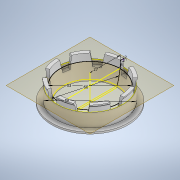
# Autodesk Inventor part: motor_frontalholder
Saved by Autodesk Inventor 2020 (Build 240168000, 168)
## iProperties
Created: 2019-08-02
Part Number: motor_frontalholder
Material: Generic
Document SubType Name: Modeling
Designer: erwin
Density: 1 g/cm^3
Appearance: Default
Author: erwin
Autodesk Inventor part; units mm, degrees
ref_plane "YZ Plane" through (0, 0, 0) normal (1, 0, 0) x (0, 1, 0)
ref_plane "XZ Plane" through (0, 0, 0) normal (0, 1, 0) x (-1, 0, 0)
ref_plane "XY Plane" through (0, 0, 0) normal (0, 0, 1) x (1, 0, 0)
sketch "Sketch1" plane through (0, 0, 0) normal (0, 1, 0) x (-1, 0, 0)
  circle A0 centre (0, 0) radius 34
  circle A1 centre (0, 0) radius 24
  dimension "d1" = 68
  dimension "d2" = 48
  constraints: 2 centre point, 1 coincident
  measures "d1" diameter of A0
  measures "d2" diameter of A1
extrude "Extrusion1" add sketch "Sketch1" along normal blind 1.5
sketch "Sketch2" plane through (0, 1.5, 0) normal (0, 1, 0) x (1, 0, 0)
  circle A0 centre (0, 0) radius 24 projected
  circle A1 centre (0, 0) radius 29
  dimension "d5" = 58
  constraints: 1 centre point, 1 coincident
  measures "d5" diameter of A1
ref_plane "Work Plane1" through (0, 13.5, 0) normal (0, 1, 0) x (1, 0, 0)
sketch "Sketch3" plane through (0, 13.5, 0) normal (0, 1, 0) x (1, 0, 0)
  circle A0 centre (0, 0) radius 29 projected
  circle A1 centre (0, 0) radius 26.5
  dimension "d7" = 53
  constraints: 1 centre point, 1 coincident
  measures "d7" diameter of A1
sketch "Sketch4" plane through (0, 0, 0) normal (1, 0, 0) x (0, 1, 0)
  line L0 (13.5, -26.5) -> (13.5, 26.5) projected
  line L1 (1.5, 24) -> (1.5, -24) projected
  line L2 (0, 24) -> (0, -24) projected
  line L3 (1.5, 24) -> (1.5, -24) projected
  arc A0 (1.5, -24) -> (19.5, -27) centre (20.2492, 32.9953) ccw
  line L4 (1.5, -29) -> (1.5, 29) projected
  line L5 (13.5, -29) -> (13.5, 29) projected
  line L6 (13.5, -29) -> (1.5, -29)
  line L7 (-3.9346, 0) -> (23.6079, 0) projected
  line L8 (13.5, -29) -> (17.5, -29)
  line L9 (17.5, -29) -> (18.5, -29.8747)
  line L10 (19.5, -29.8747) -> (19.5, -27)
  line L11 (19.5, -29.8747) -> (18.5, -29.8747)
  point P0 (0, 0)
  point P1 (13.5, -26.6239)
  dimension "d8" = 60
  dimension "d12" = 4
  dimension "d13" = 2
  dimension "d14" = 1
  dimension "d20" = 27
  constraints: 10 end point, 3 horizontal, 2 point on circle, 1 centre point, 1 perpendicular
  measures "d8" radius of A0
  measures "d12" distance of L5.start L8.end
  measures "d13" distance from line of L10 L8.end
  measures "d14" distance of L10.start L9.end
  measures "d20" distance from line of L7 L10.end
revolve "Revolution1" add sketch "Sketch4" angle 360 about axis through (0, -10, 0) along (0, 1, 0) contours L5 L6 L4 A0 | A0 L10 L11 L9 L8 L5
sketch "Sketch5" plane through (0, 0, 0) normal (1, 0, 0) x (0, 1, 0)
  line L0 (0, 34) -> (1.5, 34) projected
  line L1 (1.5, 34) -> (1.5, 29) projected
  line L2 (1.5, 29) -> (17.5, 29) projected
  line L3 (17.5, 29) -> (18.5, 29.8747) projected
  line L4 (18.5, 29.8747) -> (19.5, 29.8747) projected
  line L5 (19.5, 29.8747) -> (19.5, 27) projected
  arc A0 (19.5, 27) -> (1.5, 24) centre (20.2492, -32.9953) ccw projected
  line L6 (1.5, 24) -> (0, 24) projected
  line L7 (0, 24) -> (0, 34) projected
  line L8 (1.5, -34) -> (0, -34) projected
  line L9 (0, -34) -> (0, -24) projected
  line L10 (0, -24) -> (1.5, -24) projected
  arc A1 (1.5, -24) -> (19.5, -27) centre (20.2492, 32.9953) ccw projected
  line L11 (19.5, -27) -> (19.5, -29.8747) projected
  line L12 (19.5, -29.8747) -> (18.5, -29.8747) projected
  line L13 (18.5, -29.8747) -> (17.5, -29) projected
  line L14 (17.5, -29) -> (1.5, -29) projected
  line L15 (1.5, -29) -> (1.5, -34) projected
  line L16 (17.5, 29) -> (1.5, 29) projected
  line L17 (9.5, 29) -> (9.5, 26.0339)
  point P0 (0, 0)
  constraints: 2 end point, 1 midpoint, 1 perpendicular, 1 point on circle
revolve "Revolution2" cut sketch "Sketch5" angle 20 about axis through (0, -10, 0) along (0, -1, 0) contours L2 L3 L4 L5 A0 L17
draft "FaceDraft1" angle 10 pull direction (0, 1, 0) faces at (-9.6384, 13.2712, 26.4812) (0, 13.2712, 28.1807) fixed edges at (-9.7261, 19.5, 26.7224) (0, 19.5, 28.4373)
pattern_circular "Circular Pattern1" count 8 over 360 about axis through (0, -10, 0) along (0, 1, 0) of "Revolution2", "FaceDraft1"
sketch "Sketch6" plane through (0, 1.5, 0) normal (0, 1, 0) x (1, 0, 0)
  circle A0 centre (0, 0) radius 29.375
  circle A1 centre (0, 0) radius 29 projected
  dimension "d21" = 58.75
  constraints: 1 centre point, 1 coincident
  measures "d21" diameter of A0
extrude "Extrusion2" add sketch "Sketch6" along normal blind 12
body "Solid1"
